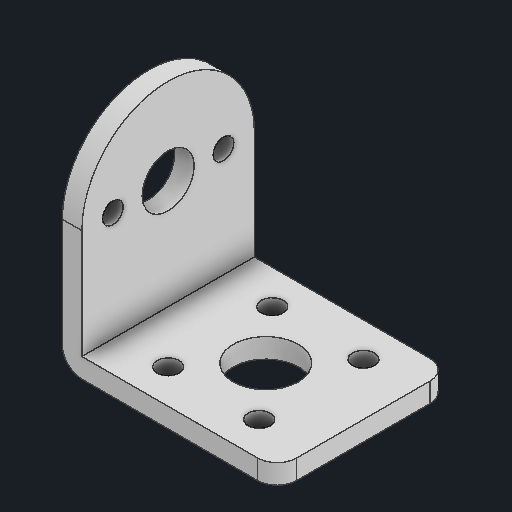
# Autodesk Inventor part: do_ga
Saved by Autodesk Inventor 2026 (Build 300175000, 175)
## iProperties
Created: 2026-08-02
Part Number: do_ga
Material: Generic
Document SubType Name: Modeling
Designer: imcle
Density: 1 g/cm^3
Appearance: Default
Author: imcle
Autodesk Inventor part; units mm, degrees
ref_plane "YZ Plane" through (0, 0, 0) normal (1, 0, 0) x (0, 1, 0)
ref_plane "XZ Plane" through (0, 0, 0) normal (0, 1, 0) x (-1, 0, 0)
ref_plane "XY Plane" through (0, 0, 0) normal (0, 0, 1) x (1, 0, 0)
sketch "Sketch1" plane through (0, 0, 0) normal (0, 0, 1) x (1, 0, 0)
  line L0 (3, 0) -> (33, 0)
  line L1 (33, 0) -> (33, 3)
  line L2 (33, 3) -> (3, 3)
  line L3 (3, 3) -> (3, 33)
  line L4 (3, 33) -> (0, 33)
  line L5 (0, 33) -> (0, 3)
  arc A0 (0, 3) -> (3, 0) centre (3, 3) ccw
  point P0 (0, 0)
  constraints: 12 end point, 2 parallel, 2 point on circle, 1 centre point, 1 coincident, 1 horizontal, 1 perpendicular
extrude "Extrusion1" add sketch "Sketch1" along normal blind 26.5
sketch "Sketch2" plane through (3, 3, 0) normal (1, 0, 0) x (0, 0, -1)
  line L0 (0, 30) -> (-26.5, 30) projected
  circle A0 centre (-13.25, 16.75) radius 13.25
  line L1 (0, 0) -> (0, 30) projected
  circle A1 centre (-13.25, 16.75) radius 4
  line L2 (-21.75, 16.75) -> (-4.75, 16.75)
  circle A2 centre (-4.75, 16.75) radius 1.6
  circle A3 centre (-21.75, 16.75) radius 1.6
  line L3 (-26.5, 0) -> (-26.5, 30) projected
  point P0 (0, -3)
  point P1 (-26.5, 16.75)
  point P2 (-13.25, 30)
  point P3 (0, 16.75)
  dimension "d9" = 3.2
  dimension "d10" = 3.2
  constraints: 4 centre point, 3 coincident, 2 end point, 1 horizontal, 1 midpoint, 1 tangent
  measures "d9" diameter of A2
  measures "d10" diameter of A3
extrude "Extrusion2" cut sketch "Sketch2" against normal up to surface (3 mm away) contours L1 A0 L0 | A0 L3 L0 | L2 A1 | A3 | A1 L2 | A2
sketch "Sketch3" plane through (3, 3, 0) normal (0, 1, 0) x (1, 0, 0)
  line L0 (30, 0) -> (30, -26.5) projected
  line L1 (30, 0) -> (0, 0) projected
  line L2 (30, -26.5) -> (0, -26.5) projected
  line L3 (30, 0) -> (27, 0)
  arc A0 (30, -3) -> (27, 0) centre (27, -3) ccw
  arc A1 (27, -26.5) -> (30, -23.5) centre (27, -23.5) ccw
  circle A2 centre (15, -13.25) radius 5
  circle A3 centre (22, -5.25) radius 1.7
  circle A4 centre (8, -5.25) radius 1.7
  circle A5 centre (22, -21.25) radius 1.7
  circle A6 centre (8, -21.25) radius 1.7
  point P0 (-3, 0)
  point P1 (30, -23.5)
  constraints: 7 centre point, 4 point on circle, 2 end point, 2 point on line
extrude "Extrusion3" cut sketch "Sketch3" against normal up to surface (3 mm away)
body "Solid1"
